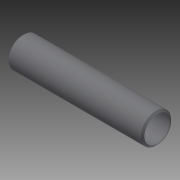
# Autodesk Inventor part: D-7516-2.75
Saved by Autodesk Inventor 2014 (Build 180170000, 170)
## iProperties
Created: 2014-01-19
Part Number: D-7516-2.75
Material: Generic
Catalog Web Link: www.cadenas.de
Description: Tube Cyl-Original Line Cyl
Vendor: BIMBA
Document SubType Name: Standard Catalog Part
Designer: Michael
Manufacturer: BIMBA
Density: 1 g/cm^3
Appearance: RGB(180.00000447034725,180.00000447034725,180.00000447034725)
Category: PARTsolutions
Company: BIMBA
Title: D-7516-2.75
Author: Cadenas PARTsolutions
Comments: Original Line Cyl
PSOL_IDENT_0: {$CADENAS_DATA\23d-libs\bimba\bimba\bimba_imperial\bimba_full_line\original_line_cylinders\three_pos
PSOL_IDENT_1: ition_cylinders\tube_cyl.prj},171 {VTYP=3D},{NB=D-7516-2.75},{LINA=D-7516-2.75},{NN=Tube Cyl},{DATE=
PSOL_IDENT_2: 14.12.2012 11:16:15},{GEOMDATE=25.01.2011 07:09:00},{VERSION=},{LINEID=60},{LINESUBID=-1},{WBVAR=MNT
PSOL_IDENT_3: ,L}  {NB=D-7516-2.75},{LINA=D-7516-2.75},{KT=DUMMY},{PN=D-7516},{MNT=},{L=2.750},{A5=0.02500000},{A5
PSOL_IDENT_4: 1=0.02500000},{B=0.61500000},{B1=0.52300000},{B2=0.57300000},{LMIN=0.130},{MIN=0.08000000},{VD=0.000
PSOL_IDENT_5: 00000},{VH=0.00000000},{A55=0.02500000},{BR=0.52260000},{CP=0.05000000},{BB=0.61500000},{BB1=0.61500
PSOL_IDENT_6: 000},{BD=0.615}
CNS_NN: Tube Cyl
CNS_NT: Original Line Cyl
CNS_NB: D-7516-2.75
CNS_NBSYN: $PN.$MNT.-$L.
CNS_LINA: D-7516-2.75
CNS_PN: D-7516
CNS_MNT: Nose Mounting
CNS_L: 2.750
CNS_A5: 0.02500000
CNS_A51: 0.02500000
CNS_B: 0.61500000
CNS_B1: 0.52300000
CNS_B2: 0.57300000
CNS_LMIN: 0.130
CNS_MIN: 0.08000000
CNS_VD: 0.00000000
CNS_VH: 0.00000000
CNS_A55: 0.02500000
CNS_BR: 0.52260000
CNS_CP: 0.05000000
CNS_BB: 0.61500000
CNS_BB1: 0.61500000
CNS_BD: 0.615
SUPPLIER: BIMBA
ARTICLENO: D-7516-2.75
BOMINFO: D-7516-2.75
CREATOR: CADENAS GmbH
Autodesk Inventor part; units mm, degrees
ref_plane "YZ Plane" through (0, 0, 0) normal (1, 0, 0) x (0, 1, 0)
ref_plane "XZ Plane" through (0, 0, 0) normal (0, 1, 0) x (-1, 0, 0)
ref_plane "XY Plane" through (0, 0, 0) normal (0, 0, 1) x (1, 0, 0)
sketch "Sketch_5" plane through (0, 0, 0) normal (0, 0, 1) x (1, 0, 0)
  line L0 (69.85, 0) -> (-69.85, 0)
  line L1 (0, 6.9051) -> (0.263, 6.6421)
  line L2 (0.263, 6.6421) -> (0.635, 6.6421)
  line L3 (0.635, 6.6421) -> (1.27, 7.2771)
  line L4 (1.27, 7.2771) -> (68.58, 7.2771)
  line L5 (68.58, 7.2771) -> (69.215, 6.6421)
  line L6 (69.215, 6.6421) -> (69.587, 6.6421)
  line L7 (69.587, 6.6421) -> (69.85, 6.9051)
  line L8 (69.85, 6.9051) -> (68.9446, 7.8105)
  line L9 (68.9446, 7.8105) -> (0.9054, 7.8105)
  line L10 (0.9054, 7.8105) -> (0, 6.9051)
  constraints: 22 end point
revolve "Revolution1" add sketch "Sketch_5" angle 360 about axis through (69.85, 0, 0) along (1, 0, 0)
ref_plane "o1_XY" through (0, -7.8105, 0) normal (1, 0, 0) x (0, 0, -1)
ref_plane "o1_YZ" through (0, -7.8105, 0) normal (0, 0, -1) x (0, 1, 0)
ref_plane "o1_ZX" through (0, -7.8105, 0) normal (0, 1, 0) x (1, 0, 0)
ref_plane "o2_XY" through (0, 7.8105, 0) normal (1, 0, 0) x (0, 0, -1)
ref_plane "o2_YZ" through (0, 7.8105, 0) normal (0, 0, -1) x (0, 1, 0)
ref_plane "o2_ZX" through (0, 7.8105, 0) normal (0, 1, 0) x (1, 0, 0)
ref_plane "t1_XY" through (34.925, 7.8105, 0) normal (1, 0, 0) x (0, 0, -1)
ref_plane "t1_YZ" through (34.925, 7.8105, 0) normal (0, 0, -1) x (0, 1, 0)
ref_plane "t1_ZX" through (34.925, 7.8105, 0) normal (0, 1, 0) x (1, 0, 0)
ref_plane "t2_XY" through (34.925, 0, -7.8105) normal (1, 0, 0) x (0, 0, -1)
ref_plane "t2_YZ" through (34.925, 0, -7.8105) normal (0, 0, -1) x (0, 1, 0)
ref_plane "t2_ZX" through (34.925, 0, -7.8105) normal (0, 1, 0) x (1, 0, 0)
ref_plane "t3_XY" through (34.925, -7.8105, 0) normal (1, 0, 0) x (0, 0, -1)
ref_plane "t3_YZ" through (34.925, -7.8105, 0) normal (0, 0, -1) x (0, 1, 0)
ref_plane "t3_ZX" through (34.925, -7.8105, 0) normal (0, 1, 0) x (1, 0, 0)
ref_plane "t4_XY" through (34.925, 0, 7.8105) normal (1, 0, 0) x (0, 0, -1)
ref_plane "t4_YZ" through (34.925, 0, 7.8105) normal (0, 0, -1) x (0, 1, 0)
ref_plane "t4_ZX" through (34.925, 0, 7.8105) normal (0, 1, 0) x (1, 0, 0)
ref_plane "tube1_XY" through (1.27, 0, 0) normal (1, 0, 0) x (0, 0, -1)
ref_plane "tube1_YZ" through (1.27, 0, 0) normal (0, 0, -1) x (0, 1, 0)
ref_plane "tube1_ZX" through (1.27, 0, 0) normal (0, 1, 0) x (1, 0, 0)
ref_plane "tube2_XY" through (68.58, 0, 0) normal (1, 0, 0) x (0, 0, -1)
ref_plane "tube2_YZ" through (68.58, 0, 0) normal (0, 0, -1) x (0, 1, 0)
ref_plane "tube2_ZX" through (68.58, 0, 0) normal (0, 1, 0) x (1, 0, 0)
body "Solid1"
